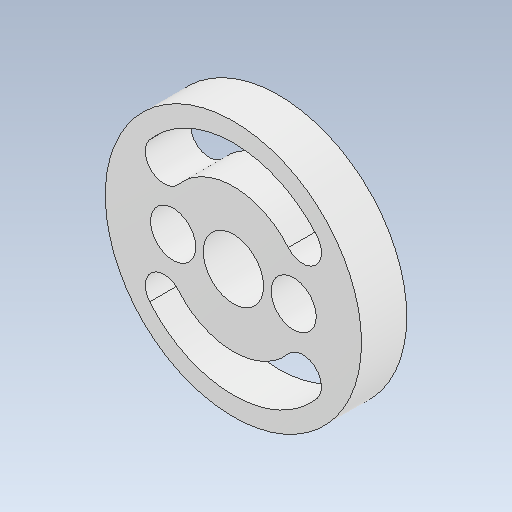
# Autodesk Inventor part: 脚中間フレームカム2
Saved by Autodesk Inventor 2020.2 (Build 242310000, 310)
## iProperties
Created: 2020-03-13
Part Number: 脚中間フレームカム2
Material: アセタール樹脂、白
Document SubType Name: Modeling
Designer: aoyam
Density: 1.425 g/cm^3
Appearance: 滑らか - 白
Mass: 0.590374 g
Surface Area: 7.03455 cm^2
Volume: 0.414298 cm^3
Author: aoyam
Autodesk Inventor part; units mm, degrees
ref_plane "YZ Plane" through (0, 0, 0) normal (1, 0, 0) x (0, 1, 0)
ref_plane "XZ Plane" through (0, 0, 0) normal (0, 1, 0) x (-1, 0, 0)
ref_plane "XY Plane" through (0, 0, 0) normal (0, 0, 1) x (1, 0, 0)
sketch "スケッチ1" plane through (0, 0, 0) normal (0, 0, 1) x (1, 0, 0)
  line L0 (0, 0) -> (-4, 0) construction
  circle A0 centre (-4, 0) radius 1.5
  line L1 (0, 0) -> (4, 0) construction
  circle A1 centre (4, 0) radius 1.5
  line L2 (0, 0) -> (0, 4.3) construction
  line L3 (0, 0) -> (-8.8388, 8.8388) construction
  circle A2 centre (-8.8388, 8.8388) radius 1.5
  line L4 (0, 0) -> (-8.8388, -8.8388) construction
  circle A3 centre (-8.8388, -8.8388) radius 1.5
  line L5 (0, 0) -> (8.8388, -8.8388) construction
  circle A4 centre (8.8388, -8.8388) radius 1.5
  line L6 (0, 0) -> (8.8388, 8.8388) construction
  circle A5 centre (8.8388, 8.8388) radius 1.5
  circle A6 centre (0, 0) radius 8.5
  circle A7 centre (0, 0) radius 15.5
  circle A8 centre (0, 0) radius 2
  dimension "d0" = 4
  dimension "d1" = 3
  dimension "d4" = 360
  dimension "d6" = 12.5
  dimension "d7" = 3
  dimension "d8" = 45
  dimension "d11" = 360
  dimension "d14" = 17
  dimension "d15" = 1.5
  dimension "d16" = 4
  constraints: 14 end point, 11 coincident, 9 centre point, 1 horizontal, 30 other
  measures "d0" distance of L0.start L0.end
  measures "d1" diameter of A0
  measures "d6" distance of L2.start L3.end
  measures "d7" diameter of A2
  measures "d8" angle of L3 L0
  measures "d14" diameter of A6
  measures "d16" diameter of A8
extrude "押し出し1" add sketch "スケッチ1" along normal blind 3 contours A6
sketch "スケッチ4" plane through (0, 0, 3) normal (0, 0, 1) x (1, 0, 0)
  circle A0 centre (0, 0) radius 8.5 projected
  circle A1 centre (-4, 0) radius 1.5 projected
  circle A2 centre (4, 0) radius 1.5 projected
  circle A3 centre (0, 0) radius 2 projected
  line L0 (0, 0) -> (-4.5963, 3.8567)
  line L1 (0, 0) -> (6, 0) construction
  line L2 (0, 0) -> (4.5963, 3.8567)
  line L3 (0, 0) -> (6, 0) construction
  arc A4 (4.5963, 3.8567) -> (-4.5963, 3.8567) centre (0, 0) ccw construction
  arc A5 (5.5538, 4.6602) -> (-5.5538, 4.6602) centre (0, 0) ccw
  arc A6 (3.6387, 3.0532) -> (-3.6387, 3.0532) centre (0, 0) ccw
  arc A7 (3.6387, 3.0532) -> (5.5538, 4.6602) centre (4.5963, 3.8567) ccw
  arc A8 (-5.5538, 4.6602) -> (-3.6387, 3.0532) centre (-4.5963, 3.8567) ccw
  line L4 (-4, 0) -> (4, 0)
  arc A9 (-5.5538, -4.6602) -> (5.5538, -4.6602) centre (0, 0) ccw
  arc A10 (-3.6387, -3.0532) -> (3.6387, -3.0532) centre (0, 0) ccw
  arc A11 (5.5538, -4.6602) -> (3.6387, -3.0532) centre (4.5963, -3.8567) ccw
  arc A12 (-3.6387, -3.0532) -> (-5.5538, -4.6602) centre (-4.5963, -3.8567) ccw
  dimension "d29" = 6
  dimension "d30" = 140
  dimension "d31" = 6
  dimension "d32" = 40
  dimension "d33" = 2.5
  constraints: 18 point on circle, 10 end point, 9 centre point, 6 symmetric about line, 4 tangent, 2 equal length, 2 horizontal, 4 other
  measures "d29" distance of L0.start L0.end
  measures "d30" angle of L1 L0
  measures "d31" distance of L0.start L2.end
  measures "d32" angle of L3 L2
  measures "d33" diameter of A7
extrude "押し出し4" cut sketch "スケッチ4" against normal blind 3 contours A8 A5 A7 A6 | A12 A10 A11 A9
